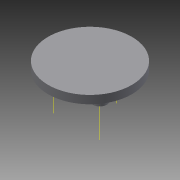
# Autodesk Inventor part: PSteg
Saved by Autodesk Inventor 2014 (Build 180170000, 170)
## iProperties
Created: 2013-05-24
Part Number: PSteg
Material: Generisch
Document SubType Name: Modeling
Designer: Felix
Density: 1 g/cm^3
Appearance: Vorgabe
Mass: 0.730568 g
Surface Area: 8.68855 cm^2
Volume: 0.730568 cm^3
Author: Felix
Autodesk Inventor part; units mm, degrees
ref_plane "YZ Plane" through (0, 0, 0) normal (1, 0, 0) x (0, 1, 0)
ref_plane "XZ Plane" through (0, 0, 0) normal (0, 1, 0) x (-1, 0, 0)
ref_plane "XY Plane" through (0, 0, 0) normal (0, 0, 1) x (1, 0, 0)
sketch "Sketch1" plane through (0, 0, 0) normal (0, 0, 1) x (1, 0, 0)
  circle A0 centre (0, 6.647) radius 1.75
  point P0 (0, 0)
  dimension "d0" = 3.5
  dimension "d1" = 6.647
  constraints: 1 centre point
  measures "d0" diameter of A0
  measures "d1" distance of A0.centre point (0, 0)
extrude "Extrusion1" add sketch "Sketch1" against normal blind 2
pattern_circular "Circular Pattern1" count 3 over 360 about axis through (0, 0, -10) along (0, 0, 1) of "Extrusion1"
sketch "Sketch3" plane through (-5.7565, -3.3235, 0) normal (0, 0, 1) x (1, 0, 0)
  circle A0 centre (5.7565, 3.3235) radius 10.3482
  circle A1 centre (5.7565, 3.3235) radius 11.0482 projected
  dimension "d13" = 0.7
  constraints: 1 centre point, 1 coincident
  measures "d13" radial gap between concentric circles of A0 A1
extrude "Extrusion3" add sketch "Sketch3" along normal blind 2 contours A0
body "Solid1"
